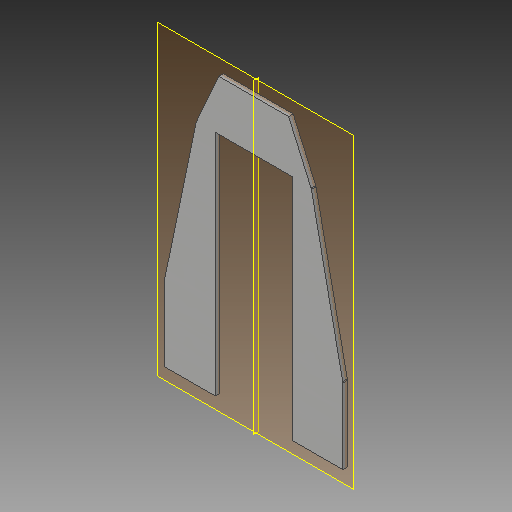
# Autodesk Inventor part: baluster-fod
Saved by Autodesk Inventor 2018 (Build 220112000, 112)
## iProperties
Created: 2019-09-28
Part Number: baluster-fod
Material: S355MC
Document SubType Name: Sheet Metal
Designer: loppen
Density: 7.85 g/cm^3
Sheet Metal Rule: Default_mm
Appearance: Light Gray
Mass: 228.91 g
Surface Area: 219.368 cm^2
Volume: 29.1606 cm^3
Flat Pattern Width: 11.6 cm
Flat Pattern Length: 18.1389 cm
Flat Pattern Area: 210.411 cm^2
Sheet Metal Width: 116,000 mm
Sheet Metal Length: 181,389 mm
Sheet Metal Area: 21041,105 mm^2
Author: loppen
Autodesk Inventor part; units mm, degrees
ref_plane "YZ Plane" through (0, 0, 0) normal (1, 0, 0) x (0, 1, 0)
ref_plane "XZ Plane" through (0, 0, 0) normal (0, 1, 0) x (-1, 0, 0)
ref_plane "XY Plane" through (0, 0, 0) normal (0, 0, 1) x (1, 0, 0)
ref_plane "Work Plane1" through (16.5341, 952.9567, 0) normal (0, 0, 1) x (-1, 0, 0)
sketch "Sketch4" plane through (16.5341, 952.9567, 3) normal (0, 0, 1) x (1, 0, 0)
  line L0 (-26.5, -89.1167) -> (-26.5, 59.6119)
  line L1 (26.5, 59.6119) -> (26.5, -89.1167)
  line L2 (-26.5, 59.6119) -> (26.5, 59.6119)
  line L3 (-25, 59.6119) -> (-25, -89.1167)
  line L4 (26.5, 59.6119) -> (-26.5, 59.6119)
  line L5 (25, 59.6119) -> (25, -89.1167)
  line L6 (-26.5, -89.1167) -> (-25, -89.1167)
  line L7 (58, -89.1167) -> (26.5, -89.1167)
  line L8 (26.5, -89.1167) -> (25, -89.1167)
  point P0 (-16.5341, -952.9567)
  dimension "d15" = 1.5
  dimension "d16" = 1.5
  measures "d15" distance between parallel lines of L0 L3
  measures "d16" distance between parallel lines of L1 L5
sketch "Sketch1" plane through (16.5341, 952.9567, 0) normal (0, 0, 1) x (-1, 0, 0)
  line L0 (60, 40.2719) -> (60, 137.1193)
  ellipse E0 centre (56, 137.1193) end of major axis (56, 141.9614) minor radius 4 (60, 137.1193) -> (56, 141.9614) ccw
  line L1 (56, 141.9614) -> (24.75, 141.9614)
  line L2 (24.75, 141.9614) -> (24.75, 144.3824)
  line L3 (24.75, 144.3824) -> (24.75, 146.8034)
  line L4 (24.75, 146.8034) -> (56, 146.8034)
  ellipse E1 centre (56, 137.1193) end of major axis (56, 146.8034) minor radius 8 (64, 137.1193) -> (56, 146.8034) ccw
  line L5 (64, 137.1193) -> (64, 40.2719)
  ellipse E2 centre (56, 40.2719) end of major axis (56, 30.5879) minor radius 8 (63.7591, 37.9134) -> (64, 40.2719) ccw
  line L6 (63.7591, 37.9134) -> (43.4204, -60.1335)
  ellipse E3 centre (35.6613, -57.775) end of major axis (35.6613, -67.459) minor radius 8 (42.7123, -62.3499) -> (43.4204, -60.1335) ccw
  line L7 (42.7123, -62.3499) -> (7.051, -142.8866)
  ellipse E4 centre (0, -138.3116) end of major axis (0, -147.9957) minor radius 8 (-7.051, -142.8866) -> (7.051, -142.8866) ccw
  line L8 (-7.051, -142.8866) -> (-42.7123, -62.3499)
  ellipse E5 centre (-35.6613, -57.775) end of major axis (-35.6613, -67.459) minor radius 8 (-43.4204, -60.1335) -> (-42.7123, -62.3499) ccw
  line L9 (-43.4204, -60.1335) -> (-63.7591, 37.9134)
  ellipse E6 centre (-56, 40.2719) end of major axis (-56, 30.5879) minor radius 8 (-64, 40.2719) -> (-63.7591, 37.9134) ccw
  line L10 (-64, 40.2719) -> (-64, 137.1193)
  ellipse E7 centre (-56, 137.1193) end of major axis (-56, 146.8034) minor radius 8 (-56, 146.8034) -> (-64, 137.1193) ccw
  line L11 (-56, 146.8034) -> (-24.75, 146.8034)
  line L12 (-24.75, 146.8034) -> (-24.75, 144.3824)
  line L13 (-24.75, 144.3824) -> (-24.75, 141.9614)
  line L14 (-24.75, 141.9614) -> (-56, 141.9614)
  ellipse E8 centre (-56, 137.1193) end of major axis (-56, 141.9614) minor radius 4 (-56, 141.9614) -> (-60, 137.1193) ccw
  line L15 (-60, 137.1193) -> (-60, 40.2719)
  ellipse E9 centre (-56, 40.2719) end of major axis (-56, 35.4299) minor radius 4 (-60, 40.2719) -> (-59.8796, 39.0927) ccw
  line L16 (-59.8796, 39.0927) -> (-39.5409, -58.9542)
  ellipse E10 centre (-35.6613, -57.775) end of major axis (-35.6613, -62.617) minor radius 4 (-39.5409, -58.9542) -> (-39.1868, -60.0624) ccw
  line L17 (-39.1868, -60.0624) -> (-3.5255, -140.5991)
  ellipse E11 centre (0, -138.3116) end of major axis (0, -143.1536) minor radius 4 (-3.5255, -140.5991) -> (3.5255, -140.5991) ccw
  line L18 (3.5255, -140.5991) -> (39.1868, -60.0624)
  ellipse E12 centre (35.6613, -57.775) end of major axis (35.6613, -62.617) minor radius 4 (39.1868, -60.0624) -> (39.5409, -58.9542) ccw
  line L19 (39.5409, -58.9542) -> (59.8796, 39.0927)
  ellipse E13 centre (56, 40.2719) end of major axis (56, 35.4299) minor radius 4 (59.8796, 39.0927) -> (60, 40.2719) ccw
  line L20 (-24.75, 141.9614) -> (24.75, 141.9614)
  line L21 (-60, 91.1167) -> (60, 91.1167)
  line L22 (-24.0389, -94.2722) -> (24.0389, -94.2722)
  line L23 (-24.5, 91.1167) -> (-24.5, -57.6119)
  line L24 (-24.5, -57.6119) -> (24.5, -57.6119)
  line L25 (24.5, -57.6119) -> (24.5, 91.1167)
  point P0 (16.5341, 952.9567)
  dimension "d0" = 49
  dimension "d1" = 120
  dimension "d2" = 35.5
  dimension "d3" = 88.0788
  dimension "d4" = 44.0394
  dimension "d5" = 101.6894
  dimension "d6" = 50.8447
  dimension "d7" = 15
  measures "d0" distance between parallel lines of L25 L23
  measures "d1" distance of L21.start L21.end
  measures "d2" distance between parallel lines of L0 L25
  measures "d3" distance of L18.start L18.end
  measures "d4" distance from line of point (0, -138.312) L22
  measures "d5" distance from line of L1 point (56, 40.272)
  measures "d6" distance between parallel lines of L21 L1
  measures "d7" distance from line of L24.end L19
extrude "Plate1" add sketch "Sketch1" along normal blind 3 contours E13 L19 E12 L18 L22 L17 E10 L16 E9 L15 L21 L23 L24 L25 L0
sketch "Sketch2" plane through (16.5341, 952.9567, 0) normal (0, 0, -1) x (-1, 0, 0)
  line L0 (60, -40.2719) -> (60, -91.1167) projected
  ellipse E0 centre (56, -40.2719) end of major axis (56, -35.4299) minor radius 4 (60, -40.2719) -> (59.8796, -39.0927) ccw projected
  line L1 (39.5409, 58.9542) -> (59.8796, -39.0927) projected
  ellipse E1 centre (35.6613, 57.775) end of major axis (35.6613, 62.617) minor radius 4 (39.5409, 58.9542) -> (39.1868, 60.0624) ccw projected
  line L2 (24.0389, 94.2722) -> (39.1868, 60.0624) projected
  line L3 (-24.0389, 94.2722) -> (24.0389, 94.2722) projected
  line L4 (-39.1868, 60.0624) -> (-24.0389, 94.2722) projected
  ellipse E2 centre (-35.6613, 57.775) end of major axis (-35.6613, 62.617) minor radius 4 (-39.1868, 60.0624) -> (-39.5409, 58.9542) ccw projected
  line L5 (-59.8796, -39.0927) -> (-39.5409, 58.9542) projected
  ellipse E3 centre (-56, -40.2719) end of major axis (-56, -35.4299) minor radius 4 (-59.8796, -39.0927) -> (-60, -40.2719) ccw projected
  line L6 (-60, -91.1167) -> (-60, -40.2719) projected
  line L7 (-24.5, -91.1167) -> (-60, -91.1167) projected
  line L8 (-24.5, 57.6119) -> (-24.5, -91.1167) projected
  line L9 (24.5, 57.6119) -> (-24.5, 57.6119) projected
  line L10 (24.5, -91.1167) -> (24.5, 57.6119) projected
  line L11 (60, -91.1167) -> (24.5, -91.1167) projected
  line L12 (-57.9212, -39.4989) -> (-37.5826, 58.548)
  line L13 (-37.3581, 59.2527) -> (-22.7372, 92.2722)
  line L14 (-22.7372, 92.2722) -> (22.7372, 92.2722)
  line L15 (22.7372, 92.2722) -> (37.3581, 59.2527)
  line L16 (37.5826, 58.548) -> (57.9212, -39.4989)
  line L17 (58, -40.2719) -> (58, -89.1167)
  line L18 (58, -89.1167) -> (26.5, -89.1167)
  line L19 (26.5, -89.1167) -> (26.5, 59.6119)
  line L20 (26.5, 59.6119) -> (-26.5, 59.6119)
  line L21 (-26.5, 59.6119) -> (-26.5, -89.1167)
  line L22 (-26.5, -89.1167) -> (-58, -89.1167)
  line L23 (-58, -89.1167) -> (-58, -40.2719)
  spline S0 degree 3 poles (-58, -40.2719) (-58, -40.0125) (-57.9739, -39.753) (-57.9212, -39.4989) knots 0 0 0 0 1 1 1 1
  spline S1 degree 3 poles (-37.5826, 58.548) (-37.5324, 58.7898) (-37.4581, 59.0268) (-37.3581, 59.2527) knots 0 0 0 0 1 1 1 1
  spline S2 degree 3 poles (37.3581, 59.2527) (37.4581, 59.0268) (37.5324, 58.7898) (37.5826, 58.548) knots 0 0 0 0 1 1 1 1
  spline S3 degree 3 poles (57.9212, -39.4989) (57.9739, -39.753) (58, -40.0125) (58, -40.2719) knots 0 0 0 0 1 1 1 1
  point P0 (16.5341, -952.9567)
  dimension "d9" = 2
  constraints: 24 end point, 7 parallel, 24 other
  measures "d9" distance between parallel lines of L6 L23
extrude "Cut1" cut sketch "Sketch2" against normal blind 3
ref_plane "midtplan" through (16.5341, 863.84, 0) normal (1, 0, 0) x (0, 0, -1)
ref_plane "modplan parallel med plade" through (16.5341, 952.9567, 1.5) normal (0, 0, 1) x (1, 0, 0)
sheet face with bend "Face2" sketch "Sketch4" thickness 3 toward (0, 0, -1) bend radius 3 relief straight relief width 3 relief depth 1.5
bend "Bend1"
equation "\"d2\" = -0.5 * d0 + 0.5 * d1"
equation "\"d4\" = 0.5 * d3"
equation "\"d6\" = 0.5 * d5"
equation "\"d10\" = Thickness"
equation "\"d16\" = d15"
equation "\"d8\" = Thickness"
equation "\"d17\" = BendRadius"
equation "\"d18\" = BendReliefWidth"
equation "\"d20\" = MinimumRemnant"
equation "\"d19\" = BendReliefDepth"
equation "\"d21\" = TransitionRadius"
equation "\"Thickness\" = pladetykkelse"
equation "\"BendRadius\" = Thickness"
equation "\"BendReliefWidth\" = Thickness"
equation "\"BendReliefDepth\" = 0.5 * Thickness"
equation "\"CornerReliefSize\" = 4 * Thickness"
equation "\"MinimumRemnant\" = 2 * Thickness"
equation "\"TransitionRadius\" = BendRadius"
equation "\"JacobiRadiusSize\" = BendRadius"
equation "\"GapSize\" = Thickness"
equation "\"pladetykkelse\" = 3"
equation "\"trappevinkel\" = 34.3deg"
equation "\"trappestifter_dia\" = 25"
equation "\"trappestifter_huldia\" = 25.8"
equation "\"trappestifter_skraa_huldia\" = 26.6"
equation "\"trappestifter_laengde\" = 228"
equation "\"perforeringsbredde\" = 6"
equation "\"perforeringshullaengde\" = 62.8"
equation "\"perforeringshullaengde_top\" = 61"
equation "\"perforeringshullaengde_bund\" = 61.6"
equation "\"perforeringsoffset\" = 8"
equation "\"perforeringsoffset_top\" = 8"
equation "\"perforeringsoffset_bund\" = 8"
equation "\"laskehul_dia\" = 13"
equation "\"balusterhul_udvidelse\" = 1"
equation "\"trinbredde\" = 1884"
body "Solid1"
